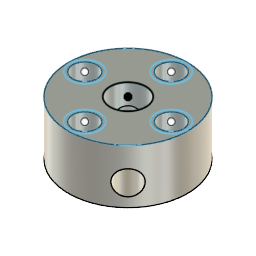
DIY7K_coupler (Autodesk Fusion 360 design; units mm, degrees)
Autodesk Fusion 360 part; units mm, degrees
sketch "スケッチ1" plane through (0, 0, 0) normal (0, 0, 1) x (1, 0, 0)
  circle A0 centre (0, 0) radius 11
  circle A1 centre (0, 8) radius 2.25
  circle A2 centre (0, 8) radius 2.75
  circle A3 centre (-8, 0) radius 2.25
  circle A4 centre (-8, 0) radius 2.75
  circle A5 centre (0, -8) radius 2.25
  circle A6 centre (0, -8) radius 2.75
  circle A7 centre (8, 0) radius 2.25
  circle A8 centre (8, 0) radius 2.75
  circle A9 centre (0, 0) radius 3.3
  dimension "d1" = 4.5
  dimension "d2" = 5.5
  dimension "d4" = 360
  dimension "d10" = 6.6
  constraint coincident A0.centre A9.centre
  constraint concentric A1 A2
  measures "d1" diameter of A1
  measures "d2" diameter of A2
  measures "d10" diameter of A9
extrude "押し出し1" add sketch "スケッチ1" against normal blind 10 contours A0 | A2 | A4 | A6 | A8 | A9
sketch "スケッチ2" plane through (0, 0, 0) normal (1, 0, 0) x (0, 1, 0)
  line L0 (0, 0) -> (0, -6)
  circle A0 through (1.591, -6, 1.591) (-0.7955, -4.0514, -0.7955) (-0.7955, -7.9486, -0.7955)
  dimension "d7" = 4.5
  constraint coincident L0.start origin
extrude "押し出し2" cut sketch "スケッチ2" against normal mid plane 32 contours A0 in plane through (0, 0, 0) normal (-0.707107, 0.707107, 0)
extrude "押し出し3" cut sketch "スケッチ1" against normal blind 10 contours A9
